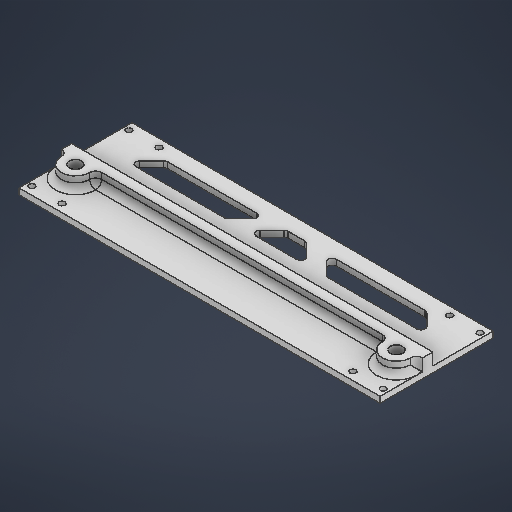
# Autodesk Inventor part: rigid_support1
Saved by Autodesk Inventor 2026.1 (Build 301233000, 233)
## iProperties
Created: 2025-10-27
Part Number: rigid_support1
Material: Generic
Document SubType Name: Modeling
Designer: emanuel
Density: 1 g/cm^3
Appearance: Default
Author: emanuel
Autodesk Inventor part; units mm, degrees
ref_plane "YZ Plane" through (0, 0, 0) normal (1, 0, 0) x (0, 1, 0)
ref_plane "XZ Plane" through (0, 0, 0) normal (0, 1, 0) x (-1, 0, 0)
ref_plane "XY Plane" through (0, 0, 0) normal (0, 0, 1) x (1, 0, 0)
sketch "Sketch1" plane through (0, 0, 0) normal (0, 1, 0) x (-1, 0, 0)
  line L0 (0, 0) -> (15, 0)
  line L1 (15, 0) -> (15, -48.3)
  line L2 (15, -48.3) -> (0, -48.3)
  line L3 (0, -48.3) -> (0, 0)
  circle A0 centre (15, 0) radius 1.5
  circle A1 centre (0, 0) radius 1.5
  circle A2 centre (15, -48.3) radius 1.5
  circle A3 centre (0, -48.3) radius 1.5
  line L4 (15, 0) -> (17.5, 0)
  line L5 (17.5, 0) -> (17.5, 4)
  line L6 (17.5, 4) -> (15, 4)
  line L7 (15, 4) -> (15, 0)
  line L8 (0, -48.3) -> (-2.5, -48.3)
  line L9 (-2.5, -48.3) -> (-2.5, -52.3)
  line L10 (-2.5, -52.3) -> (0, -52.3)
  line L11 (0, -52.3) -> (0, -48.3)
  line L12 (-2.5, -52.3) -> (17.5, -52.3)
  line L13 (17.5, -52.3) -> (17.5, 4)
  line L14 (17.5, 4) -> (-2.5, 4)
  line L15 (-2.5, 4) -> (-2.5, -52.3)
  line L16 (17.5, 4) -> (-47.5, 4)
  line L17 (-47.5, 4) -> (-47.5, -26)
  line L18 (-47.5, -26) -> (17.5, -26)
  line L19 (17.5, -26) -> (17.5, 4)
  circle A4 centre (-47.5, -26) radius 1.5
  line L20 (17.5, 4) -> (-72.5, 4)
  line L21 (17.5, 4) -> (-72.5, 4)
  line L22 (-72.5, 4) -> (-72.5, -44.8)
  line L23 (-72.5, -44.8) -> (17.5, -44.8)
  line L24 (17.5, -44.8) -> (17.5, 4)
  line L25 (-47.5, -26) -> (-57.5, -26)
  line L26 (-57.5, -26) -> (-67.5, -26)
  circle A5 centre (-67.5, -26) radius 1.5
  circle A6 centre (-57.5, -26) radius 1.5
  line L27 (-2.5, -52.3) -> (-72.5, -52.3)
  line L28 (-72.5, -52.3) -> (-72.5, -44.8)
  line L29 (-72.5, -44.8) -> (-2.5, -44.8)
  line L30 (-2.5, -44.8) -> (-2.5, -52.3)
  line L31 (-145, 0) -> (-160, 0)
  line L32 (-160, 0) -> (-160, -48.3)
  line L33 (-160, -48.3) -> (-145, -48.3)
  line L34 (-145, -48.3) -> (-145, 0)
  circle A7 centre (-160, 0) radius 1.5
  circle A8 centre (-145, 0) radius 1.5
  circle A9 centre (-160, -48.3) radius 1.5
  circle A10 centre (-145, -48.3) radius 1.5
  line L35 (-160, 0) -> (-162.5, 0)
  line L36 (-162.5, 0) -> (-162.5, 4)
  line L37 (-162.5, 4) -> (-160, 4)
  line L38 (-160, 4) -> (-160, 0)
  line L39 (-145, -48.3) -> (-142.5, -48.3)
  line L40 (-142.5, -48.3) -> (-142.5, -52.3)
  line L41 (-142.5, -52.3) -> (-145, -52.3)
  line L42 (-145, -52.3) -> (-145, -48.3)
  line L43 (-142.5, -52.3) -> (-162.5, -52.3)
  line L44 (-162.5, -52.3) -> (-162.5, 4)
  line L45 (-162.5, 4) -> (-142.5, 4)
  line L46 (-142.5, 4) -> (-142.5, -52.3)
  line L47 (-162.5, 4) -> (-97.5, 4)
  line L48 (-97.5, 4) -> (-97.5, -26)
  line L49 (-97.5, -26) -> (-162.5, -26)
  line L50 (-162.5, -26) -> (-162.5, 4)
  circle A11 centre (-97.5, -26) radius 1.5
  line L51 (-162.5, 4) -> (-72.5, 4)
  line L52 (-162.5, 4) -> (-72.5, 4)
  line L53 (-72.5, -44.8) -> (-162.5, -44.8)
  line L54 (-162.5, -44.8) -> (-162.5, 4)
  line L55 (-97.5, -26) -> (-87.5, -26)
  line L56 (-87.5, -26) -> (-77.5, -26)
  circle A12 centre (-77.5, -26) radius 1.5
  circle A13 centre (-87.5, -26) radius 1.5
  line L57 (-142.5, -52.3) -> (-72.5, -52.3)
  line L58 (-72.5, -44.8) -> (-142.5, -44.8)
  line L59 (-142.5, -44.8) -> (-142.5, -52.3)
  point P0 (0, -52.3)
  point P1 (-2.5, -46.3)
  point P2 (16.5, 0)
  point P3 (15, 1.5)
  dimension "d0" = 15
  dimension "d1" = 48.3
  dimension "d2" = 3
  dimension "d3" = 3
  dimension "d4" = 3
  dimension "d5" = 3
  dimension "d6" = 2.5
  dimension "d7" = 4
  dimension "d8" = 2.5
  dimension "d9" = 4
  dimension "d12" = 3
  dimension "d14" = 10
  dimension "d15" = 10
  dimension "d18" = 3
  dimension "d19" = 3
  dimension "d53" = 30
  constraints: 120 end point, 26 symmetric about line, 14 centre point, 14 coincident, 14 parallel, 8 horizontal, 8 perpendicular, 2 point on line, 7 other
  measures "d0" distance of L1.end L2.end
  measures "d1" distance of L0.end L1.end
  measures "d2" diameter of A0
  measures "d3" diameter of A1
  measures "d4" diameter of A2
  measures "d5" diameter of A3
  measures "d6" distance of L6.end L5.end
  measures "d7" distance of L5.end L4.end
  measures "d8" distance of L10.end L9.end
  measures "d9" distance of L9.end L8.end
  measures "d12" diameter of A4
  measures "d14" distance of L25.start L25.end
  measures "d15" distance of L25.end L26.end
  measures "d18" diameter of A5
  measures "d19" diameter of A6
  measures "d53" distance of L16.end L17.end
extrude "Extrusion1" add sketch "Sketch1" along normal blind 3 contours A1 L3 L18 L15 L14 L7 A0 L0 | L0 A0 L1 L18 L3 A1 | L18 L1 L23 L3 | L3 L23 L15 L18 | L7 L6 L5 L4 A0 | A0 L4 L13 L18 L1 | L23 L1 A2 L2 A3 L3 | L3 A3 L8 L15 L23 | L18 A4 L17 L16 L15 | L15 L23 L22 L20 L17 A4 L18 | L18 L13 L23 L1 | L15 L9 L27 L28 L23 | L23 L13 L12 L11 A3 L2 A2 L1 | A3 L11 L10 L9 L8 | L53 L46 L49 A11 L48 L51 L22 | L28 L57 L40 L46 L53 | L53 L34 L49 L46 | L46 L39 A10 L34 L53 | L48 A11 L49 L46 L47 | L41 L42 A10 L39 L40 | L49 L34 A8 L31 A7 L38 L45 L46 | L53 L32 L49 L34 | L34 A10 L33 A9 L32 L53 | L43 L44 L53 L32 A9 L33 A10 L42 | L49 L32 A7 L31 A8 L34 | L53 L44 L49 L32 | L38 A7 L35 L36 L37 | L49 L44 L35 A7 L32
sketch "Sketch4" plane through (0, 3, 0) normal (0, 1, 0) x (1, 0, 0)
  line L0 (-17.5, -4) -> (162.5, -4) projected
  line L1 (-17.5, -4) -> (-7.5, -4)
  line L2 (-7.5, -4) -> (-7.5, 14.15)
  line L3 (-7.5, 14.15) -> (-17.5, 14.15)
  line L4 (-17.5, 14.15) -> (-17.5, -4)
  line L5 (162.5, -4) -> (162.5, 52.3) projected
  line L6 (162.5, -4) -> (152.5, -4)
  line L7 (152.5, -4) -> (152.5, 14.15)
  line L8 (152.5, 14.15) -> (162.5, 14.15)
  line L9 (162.5, 14.15) -> (162.5, -4)
  circle A0 centre (152.5, 14.15) radius 3.1
  circle A1 centre (152.5, 14.15) radius 7
  circle A2 centre (-7.5, 14.15) radius 3.1
  circle A3 centre (-7.5, 14.15) radius 7
  line L10 (-7.5, 17.25) -> (-17.5, 17.25)
  line L11 (-17.5, 17.25) -> (162.5, 17.25)
  line L12 (162.5, 17.25) -> (162.5, 22.25)
  line L13 (162.5, 22.25) -> (-17.5, 22.25)
  line L14 (-17.5, 22.25) -> (-17.5, 17.25)
  point P0 (0, 0)
  point P1 (158.7761, 17.25)
  point P2 (162.5, 17.25)
  point P3 (162.5, 22.25)
  point P4 (-13.7761, 17.25)
  point P5 (-1.2239, 17.25)
  point P6 (146.2239, 17.25)
  dimension "d60" = 6.2
  dimension "d54" = 10
  dimension "d55" = 18.15
  dimension "d56" = 10
  dimension "d57" = 18.15
  dimension "d58" = 6.2
  dimension "d59" = 14
  dimension "d61" = 14
  dimension "d62" = 180
  dimension "d65" = 5
  constraints: 26 end point, 6 parallel, 5 horizontal, 4 coincident, 3 centre point, 3 perpendicular, 1 vertical alignment, 2 other
  measures "d54" distance of L3.end L2.end
  measures "d55" distance of L2.end L1.end
  measures "d56" distance of L7.end L8.end
  measures "d57" distance of L6.end L7.end
  measures "d58" diameter of A0
  measures "d59" diameter of A1
  measures "d61" diameter of A3
  measures "d62" distance of L13.end L12.end
  measures "d65" distance between parallel lines of L13 L11
extrude "Extrusion4" add sketch "Sketch4" along normal blind 6 contours A3 L3 A2 L2 | L2 A2 L11 A3 | A3 L10 A2 L3 | A1 L11 A0 L7 | L7 A0 L8 A1 | L10 L14 L13 L5 L11 A1 A3 | A3 L11 L10 | A1 L11 | L8 A0 L11 A1
fillet "Fillet5" radius 3 7 edges at (72.5, 3, -17.25) (-7.5, 3, -7.15) (-13.7761, 6, -17.25) (-1.2239, 6, -17.25) (146.2239, 6, -17.25) (152.5, 3, -7.15) (158.7761, 6, -17.25)
sketch "Sketch5" plane through (0, 3, 0) normal (0, 1, 0) x (1, 0, 0)
  line L0 (162.5, 52.3) -> (-17.5, 52.3) projected
  line L1 (-17.5, 52.3) -> (7.5, 52.3)
  line L2 (7.5, 52.3) -> (7.5, 44.3)
  line L3 (7.5, 44.3) -> (-17.5, 44.3)
  line L4 (-17.5, 44.3) -> (-17.5, 52.3)
  line L5 (162.5, 22.25) -> (162.5, 52.3) projected
  line L6 (162.5, 52.3) -> (137.5, 52.3)
  line L7 (137.5, 52.3) -> (137.5, 44.3)
  line L8 (137.5, 44.3) -> (162.5, 44.3)
  line L9 (162.5, 44.3) -> (162.5, 52.3)
  line L10 (7.5, 44.3) -> (47.5, 44.3)
  line L11 (47.5, 44.3) -> (47.5, 34.3)
  line L12 (47.5, 34.3) -> (7.5, 34.3)
  line L13 (7.5, 34.3) -> (7.5, 44.3)
  line L14 (137.5, 44.3) -> (97.5, 44.3)
  line L15 (97.5, 44.3) -> (97.5, 34.3)
  line L16 (97.5, 34.3) -> (137.5, 34.3)
  line L17 (137.5, 34.3) -> (137.5, 44.3)
  line L18 (47.5, 44.3) -> (57.5, 44.3)
  line L19 (57.5, 44.3) -> (47.5, 34.3)
  line L20 (97.5, 44.3) -> (87.5, 44.3)
  line L21 (87.5, 44.3) -> (97.5, 34.3)
  line L22 (137.5, 34.3) -> (147.5, 34.3)
  line L23 (7.5, 34.3) -> (-2.5, 34.3)
  line L24 (-2.5, 34.3) -> (7.5, 44.3)
  line L25 (137.5, 44.3) -> (147.5, 34.3)
  line L26 (57.5, 44.3) -> (67.5, 44.3)
  line L27 (87.5, 44.3) -> (77.5, 44.3)
  line L28 (77.5, 44.3) -> (67.5, 44.3)
  line L29 (47.5, 34.3) -> (57.5, 34.3)
  line L30 (57.5, 34.3) -> (87.5, 34.3)
  line L31 (87.5, 34.3) -> (77.5, 44.3)
  line L32 (67.5, 44.3) -> (57.5, 34.3)
  point P0 (0, 0)
  dimension "d67" = 25
  dimension "d68" = 8
  dimension "d69" = 25
  dimension "d70" = 8
  dimension "d71" = 40
  dimension "d72" = 10
  dimension "d73" = 40
  dimension "d74" = 10
  dimension "d75" = 10
  dimension "d76" = 10
  dimension "d77" = 10
  dimension "d78" = 10
  dimension "d82" = 10
  dimension "d83" = 10
  dimension "d84" = 10
  dimension "d85" = 30
  constraints: 62 end point, 9 parallel, 8 horizontal, 6 perpendicular, 5 point on line
  measures "d67" distance of L2.end L3.end
  measures "d68" distance of L1.end L2.end
  measures "d69" distance of L8.end L7.end
  measures "d70" distance of L7.end L6.end
  measures "d71" distance of L11.end L12.end
  measures "d72" distance of L10.end L11.end
  measures "d73" distance of L16.end L15.end
  measures "d74" distance of L15.end L14.end
  measures "d75" distance of L10.end L18.end
  measures "d76" distance of L14.end L20.end
  measures "d77" distance of L16.end L22.end
  measures "d78" distance of L12.end L23.end
  measures "d82" distance of L18.end L26.end
  measures "d83" distance of L20.end L27.end
  measures "d84" distance of L11.end L29.end
  measures "d85" distance of L29.end L30.end
extrude "Extrusion5" cut sketch "Sketch5" against normal blind 6 contours L17 L16 L15 L14 | L25 L22 L17 | L10 L11 L12 L13 | L13 L23 L24 | L15 L21 L20 | L18 L19 L11 | L31 L30 L32 L28
fillet "Fillet6" radius 2 12 edges at (7.5, 1.5, -44.3) (-2.5, 1.5, -34.3) (57.5, 1.5, -44.3) (47.5, 1.5, -34.3) (87.5, 1.5, -44.3) (97.5, 1.5, -34.3) (147.5, 1.5, -34.3) (137.5, 1.5, -44.3) (67.5, 1.5, -44.3) (77.5, 1.5, -44.3) (87.5, 1.5, -34.3) (57.5, 1.5, -34.3)
body "Solid1"
